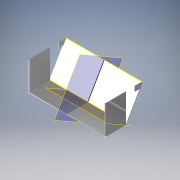
# Autodesk Inventor part: 15102898-16-P-0203
Saved by Autodesk Inventor 2017 (Build 210142000, 142)
## iProperties
Created: 2016-10-01
Part Number: 15102898-16-P-0203
Material: Polycarbonate, Clear
Document SubType Name: Modeling
Designer: Sofia
Density: 1.2 g/cm^3
Appearance: Polycarbonate - Clear
Author: Sofia
Autodesk Inventor part; units mm, degrees
ref_plane "YZ Plane" through (0, 0, 0) normal (1, 0, 0) x (0, 1, 0)
ref_plane "XZ Plane" through (0, 0, 0) normal (0, 1, 0) x (-1, 0, 0)
ref_plane "XY Plane" through (0, 0, 0) normal (0, 0, 1) x (1, 0, 0)
sketch "Sketch1" plane through (0, 0, 0) normal (0, 1, 0) x (-1, 0, 0)
  line L0 (0, 0) -> (-415.7726, 0)
  line L1 (-415.7726, 0) -> (-415.7726, -115.7143)
  line L2 (-415.7726, -115.7143) -> (0, -115.7143)
  line L3 (0, -115.7143) -> (0, 0)
  dimension "d0" = 415.7726
  constraints: 8 end point, 2 parallel, 1 horizontal, 1 perpendicular
  measures "d0" distance of L2.end L1.end
extrude "Extrusion1" add sketch "Sketch1" along normal blind 3.175
sketch "Sketch2" plane through (0, 3.175, 0) normal (0, 1, 0) x (1, 0, 0)
  line L0 (0, 0) -> (415.7726, 0) projected
  line L1 (3.175, 0) -> (3.175, 112.5393)
  line L2 (3.175, 112.5393) -> (412.5976, 112.5393)
  line L3 (412.5976, 112.5393) -> (412.5976, 0)
  line L4 (415.7726, 0) -> (415.7726, 115.7143) projected
  line L5 (0, 115.7143) -> (0, 0) projected
  line L6 (415.7726, 115.7143) -> (0, 115.7143) projected
  line L7 (0, 0) -> (3.175, 0)
  line L8 (415.7726, 0) -> (412.5976, 0)
  line L9 (3.175, 112.5393) -> (0, 112.5393)
  line L10 (412.5976, 112.5393) -> (415.7726, 112.5393)
  dimension "d3" = 3.175
  dimension "d4" = 3.175
  dimension "d5" = 3.175
  constraints: 14 end point, 4 point on line, 3 perpendicular, 2 collinear, 1 vertical
  measures "d3" distance between parallel lines of L4 L3
  measures "d4" distance between parallel lines of L1 L5
  measures "d5" distance between parallel lines of L6 L2
extrude "Extrusion6" add sketch "Sketch2" along normal blind 152.4 contours L5 L9 L1 L0 | L3 L10 L4 L0
ref_plane "Work Plane1" through (415.7726, 3.175, -115.7143) normal (0, 0.8660254, -0.5) x (-1, 0, 0)
sketch "Sketch9" plane through (415.7726, 3.175, -115.7143) normal (0, 0.8660254, -0.5) x (-1, 0, 0)
  line L0 (0, 98.6241) -> (0, -1.5875) projected
  line L1 (415.7726, 0) -> (0, 0)
  line L2 (0, 0) -> (0, 3.175)
  line L3 (0, 3.175) -> (415.7726, 3.175)
  line L4 (415.7726, 3.175) -> (415.7726, 0)
  point P0 (415.7726, 98.6241)
  dimension "d25" = 3.175
  constraints: 8 end point, 2 parallel, 1 coincident, 1 horizontal, 1 perpendicular, 1 point on line
  measures "d25" distance between parallel lines of L3 L1
extrude "Extrusion7" add sketch "Sketch9" along normal blind 175.9712
sketch "Sketch11" plane through (415.7726, 3.175, -115.7143) normal (1, 0, 0) x (0, -0.5, -0.8660254)
  point P0 (-98.6241, -60.6068)
sketch "Sketch12" plane through (415.7726, 3.175, -115.7143) normal (1, 0, 0) x (0, -0.5, -0.8660254)
  line L0 (-3.175, 175.9712) -> (-37.872, 155.9389)
  line L1 (-37.872, 155.9389) -> (-25.172, 133.9418)
  line L2 (-25.172, 133.9418) -> (-3.175, 146.6418)
  line L3 (-3.175, 0) -> (-3.175, 175.9712) projected
  point P0 (-98.6241, -60.6068)
  dimension "d34" = 25.4
  dimension "d35" = 60
  dimension "d36" = 25.4
  constraints: 6 end point, 1 parallel, 1 perpendicular, 1 point on line
  measures "d34" distance of L0.end L1.end
  measures "d35" angle of L3 L0
  measures "d36" distance of L1.end L2.end
extrude "Extrusion9" add sketch "Sketch12" against normal blind 3.175
sketch "Sketch13" plane through (0, 4.7625, -112.9647) normal (0, 0.5, 0.8660254) x (1, 0, 0)
  line L0 (415.7726, 175.9712) -> (0, 175.9712) projected
  line L1 (207.8863, 175.9712) -> (207.8863, 0)
  line L2 (415.7726, 0) -> (0, 0) projected
  point P0 (0, -60.6068)
  constraints: 2 end point, 2 midpoint
ref_plane "Work Plane2" through (207.8863, 157.158, -200.9503) normal (-1, 0, 0) x (0, -0.8660254, 0.5)
mirror "Mirror1" about plane through (207.8863, 157.158, -200.9503) normal (-1, 0, 0) of "Extrusion9"
body "Solid1"
